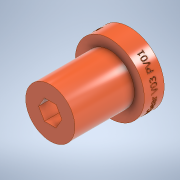
# Autodesk Inventor part: hexBushingForSideOppositeWormGear
Saved by Autodesk Inventor 2022.2 (Build 262287010, 287A)
## iProperties
Created: 2020-11-16
Part Number: hexBushingForSideOppositeWormGear
Material: PC/ABS Plastic
Document SubType Name: Modeling
Designer: robst
Density: 0.357273 g/cm^3
Appearance: Smooth - Light Orange
Author: robst
Autodesk Inventor part; units mm, degrees
(part 1 of 2)
ref_plane "YZ Plane" through (0, 0, 0) normal (1, 0, 0) x (0, 1, 0)
ref_plane "XY Plane" through (0, 0, 0) normal (0, 0, 1) x (1, 0, 0)
sketch "Sketch1" plane through (0, 0, 0) normal (0, 0, 1) x (1, 0, 0)
  line L0 (7.3323, 0) -> (3.6662, -6.35)
  line L1 (3.6662, -6.35) -> (-3.6662, -6.35)
  line L2 (-3.6662, -6.35) -> (-7.3323, 0)
  line L3 (-7.3323, 0) -> (-3.6662, 6.35)
  line L4 (-3.6662, 6.35) -> (3.6662, 6.35)
  line L5 (3.6662, 6.35) -> (7.3323, 0)
  point P0 (0, 0)
  point P1 (0, 0)
  dimension "d0" = 12.7
  constraints: 12 end point, 1 coincident, 1 horizontal, 13 other
  measures "d0" distance between parallel lines of L1 L4
extrude "Extrusion1" add sketch "Sketch1" along normal mid plane 25.4
sketch "Sketch2" plane through (0, 0, -12.7) normal (0, 0, -1) x (-1, 0, 0)
  circle A0 centre (0, 0) radius 15.748
  dimension "d3" = 31.496
  constraints: 1 centre point, 1 coincident
  measures "d3" diameter of A0
extrude "Extrusion2" add sketch "Sketch2" along normal blind 19.05
sketch "Sketch3" plane through (0, 0, -31.75) normal (0, 0, -1) x (-1, 0, 0)
  circle A0 centre (0, 0) radius 22.098
  dimension "d6" = 44.196
  constraints: 1 centre point, 1 coincident
  measures "d6" diameter of A0
extrude "Base" add sketch "Sketch3" along normal blind 12.7
sketch "Sketch6" plane through (-3.6662, 6.35, 12.7) normal (0, 1, 0) x (1, 0, 0)
  line L0 (7.3323, 0) -> (0, 0) construction
  line L1 (3.6662, 0) -> (3.6662, 34.6111) construction
  line L2 (19.4142, 25.4) -> (-12.0818, 25.4) projected
  point P0 (3.6662, 12.7)
  point P1 (3.6662, 19.2024)
  dimension "d13" = 6.1976
  constraints: 2 end point, 1 midpoint, 1 point on line, 1 vertical
  measures "d13" distance from line of point (3.666, 19.202) L2
hole "Hole1" at (0, 6.35, -6.5024) direction (0, -1, 0) diameter 4.318 end through all clearance for "Hex Machine Screw" size "#6" standard "Ansi Unified Screw Threads"
sketch "Sketch7" plane through (0, 0, 12.7) normal (0, 0, 1) x (1, 0, 0)
  point P0 (0, 0)
  point P1 (0, 0)
  constraints: 1 coincident
hole "Hole2" at (0, 0, 12.7) direction (0, 0, -1) diameter 6.3246 depth 7.874 counterbore diameter 6.604 counterbore depth 6.1239
ref_plane "Work Plane1" through (0, -22.098, -31.75) normal (0, 1, 0) x (-1, 0, 0)
sketch "Sketch8" plane through (0, -22.098, -31.75) normal (0, 1, 0) x (-1, 0, 0)
  line L0 (-22.098, -12.7) -> (22.098, -12.7) projected
  line L1 (-22.098, 0) -> (22.098, 0) projected
  line L2 (22.098, 0) -> (22.098, -12.7) construction
  line L3 (22.098, -6.35) -> (-22.098, -6.35) construction
  line L4 (-22.098, 0) -> (-22.098, -12.7) construction
  line L5 (53.7985, -8.255) -> (54.2802, -8.255)
  line L6 (54.2802, -8.255) -> (54.2802, -6.6248)
  spline S0 degree 2 poles (54.2802, -6.6248) (54.2802, -6.4272) (54.3172, -6.0876) (54.3728, -5.9857) knots 0 0 0 1 2 2 2
  spline S1 degree 2 poles (54.3728, -5.9857) (54.4314, -5.8776) (54.6414, -5.7726) (54.8205, -5.7726) knots 0 0 0 1 2 2 2
  spline S2 degree 2 poles (54.8205, -5.7726) (54.9995, -5.7726) (55.3793, -5.9641) (55.5615, -6.1184) knots 0 0 0 1 2 2 2
  line L7 (55.5615, -6.1184) -> (55.5615, -8.255)
  line L8 (55.5615, -8.255) -> (56.0431, -8.255)
  line L9 (56.0431, -8.255) -> (56.0431, -4.2752)
  line L10 (56.0431, -4.2752) -> (55.5615, -4.2752)
  line L11 (55.5615, -4.2752) -> (55.5615, -5.714)
  spline S3 degree 2 poles (55.5615, -5.714) (55.3453, -5.5195) (54.9285, -5.3157) (54.6939, -5.3157) knots 0 0 0 1 2 2 2
  spline S4 degree 2 poles (54.6939, -5.3157) (54.274, -5.3157) (53.7985, -5.8714) (53.7985, -6.3994) knots 0 0 0 1 2 2 2
  line L12 (53.7985, -6.3994) -> (53.7985, -8.255)
  spline S5 degree 2 poles (51.8811, -8.3198) (52.5666, -8.3198) (53.3199, -7.551) (53.3199, -6.8409) knots 0 0 0 1 2 2 2
  spline S6 degree 2 poles (53.3199, -6.8409) (53.3199, -6.1431) (52.5882, -5.3157) (51.9985, -5.3157) knots 0 0 0 1 2 2 2
  spline S7 degree 2 poles (51.9985, -5.3157) (51.7329, -5.3157) (51.3223, -5.4701) (51.171, -5.6337) knots 0 0 0 1 2 2 2
  spline S8 degree 2 poles (51.171, -5.6337) (51.0166, -5.7973) (50.853, -6.2697) (50.853, -6.6124) knots 0 0 0 1 2 2 2
  line L13 (50.853, -6.6124) -> (50.853, -6.8749)
  line L14 (50.853, -6.8749) -> (52.8321, -6.8749)
  spline S9 degree 2 poles (52.8321, -6.8749) (52.8321, -7.372) (52.3319, -7.8999) (51.8873, -7.8999) knots 0 0 0 1 2 2 2
  spline S10 degree 2 poles (51.8873, -7.8999) (51.7299, -7.8999) (51.4242, -7.8289) (51.3007, -7.7733) knots 0 0 0 1 2 2 2
  spline S11 degree 2 poles (51.3007, -7.7733) (51.171, -7.7116) (50.9919, -7.6035) (50.9333, -7.5541) knots 0 0 0 1 2 2 2
  line L15 (50.9333, -7.5541) -> (50.9055, -7.5541)
  line L16 (50.9055, -7.5541) -> (50.9055, -8.079)
  spline S12 degree 2 poles (50.9055, -8.079) (50.9889, -8.113) (51.242, -8.2118) (51.3408, -8.2396) knots 0 0 0 1 2 2 2
  spline S13 degree 2 poles (51.3408, -8.2396) (51.4798, -8.2797) (51.7082, -8.3198) (51.8811, -8.3198) knots 0 0 0 1 2 2 2
  spline S14 degree 2 poles (51.3223, -6.5075) (51.3285, -6.3129) (51.4088, -6.0289) (51.4859, -5.9332) knots 0 0 0 1 2 2 2
  spline S15 degree 2 poles (51.4859, -5.9332) (51.5693, -5.8251) (51.8317, -5.7109) (52.0263, -5.7109) knots 0 0 0 1 2 2 2
  spline S16 degree 2 poles (52.0263, -5.7109) (52.2177, -5.7109) (52.4863, -5.8251) (52.5975, -5.9363) knots 0 0 0 1 2 2 2
  spline S17 degree 2 poles (52.5975, -5.9363) (52.7055, -6.0505) (52.8167, -6.3253) (52.8321, -6.5075) knots 0 0 0 1 2 2 2
  line L17 (52.8321, -6.5075) -> (51.3223, -6.5075)
  line L18 (48.1452, -8.255) -> (48.735, -8.255)
  line L19 (48.735, -8.255) -> (49.4297, -7.1805)
  line L20 (49.4297, -7.1805) -> (50.1429, -8.255)
  line L21 (50.1429, -8.255) -> (50.6894, -8.255)
  line L22 (50.6894, -8.255) -> (49.6983, -6.8378)
  line L23 (49.6983, -6.8378) -> (50.6801, -5.396)
  line L24 (50.6801, -5.396) -> (50.0904, -5.396)
  line L25 (50.0904, -5.396) -> (49.3988, -6.4612)
  line L26 (49.3988, -6.4612) -> (48.6917, -5.396)
  line L27 (48.6917, -5.396) -> (48.1452, -5.396)
  line L28 (48.1452, -5.396) -> (49.1302, -6.807)
  line L29 (49.1302, -6.807) -> (48.1452, -8.255)
  spline S18 degree 2 poles (45.1504, -7.0848) (45.1504, -7.3689) (45.3665, -7.8042) (45.5456, -7.9462) knots 0 0 0 1 2 2 2
  spline S19 degree 2 poles (45.5456, -7.9462) (45.7617, -8.113) (46.2526, -8.255) (46.6416, -8.255) knots 0 0 0 1 2 2 2
  line L30 (46.6416, -8.255) -> (47.7346, -8.255)
  line L31 (47.7346, -8.255) -> (47.7346, -4.445)
  line L32 (47.7346, -4.445) -> (46.725, -4.445)
  spline S20 degree 2 poles (46.725, -4.445) (46.3174, -4.445) (45.9099, -4.4975) (45.7246, -4.5994) knots 0 0 0 1 2 2 2
  spline S21 degree 2 poles (45.7246, -4.5994) (45.5178, -4.7074) (45.3294, -5.0625) (45.3294, -5.3033) knots 0 0 0 1 2 2 2
  spline S22 degree 2 poles (45.3294, -5.3033) (45.3294, -5.5719) (45.6135, -5.998) (45.8636, -6.1184) knots 0 0 0 1 2 2 2
  line L33 (45.8636, -6.1184) -> (45.8636, -6.137)
  spline S23 degree 2 poles (45.8636, -6.137) (45.5239, -6.2296) (45.1504, -6.7205) (45.1504, -7.0848) knots 0 0 0 1 2 2 2
  spline S24 degree 2 poles (45.6783, -7.1064) (45.6783, -6.8903) (45.8018, -6.6124) (45.9871, -6.5136) knots 0 0 0 1 2 2 2
  spline S25 degree 2 poles (45.9871, -6.5136) (46.1075, -6.4519) (46.3915, -6.4148) (46.654, -6.4148) knots 0 0 0 1 2 2 2
  line L34 (46.654, -6.4148) -> (47.2283, -6.4148)
  line L35 (47.2283, -6.4148) -> (47.2283, -7.8227)
  line L36 (47.2283, -7.8227) -> (46.8176, -7.8227)
  spline S26 degree 2 poles (46.8176, -7.8227) (46.4842, -7.8227) (46.1013, -7.761) (45.9531, -7.6622) knots 0 0 0 1 2 2 2
  spline S27 degree 2 poles (45.9531, -7.6622) (45.8111, -7.5603) (45.6783, -7.3071) (45.6783, -7.1064) knots 0 0 0 1 2 2 2
  spline S28 degree 2 poles (45.8574, -5.3743) (45.8574, -5.2385) (45.95, -5.0347) (46.0519, -4.9761) knots 0 0 0 1 2 2 2
  spline S29 degree 2 poles (46.0519, -4.9761) (46.1754, -4.9081) (46.4749, -4.8773) (46.7435, -4.8773) knots 0 0 0 1 2 2 2
  line L37 (46.7435, -4.8773) -> (47.2283, -4.8773)
  line L38 (47.2283, -4.8773) -> (47.2283, -5.9918)
  line L39 (47.2283, -5.9918) -> (46.654, -5.9918)
  spline S30 degree 2 poles (46.654, -5.9918) (46.4162, -5.9918) (46.1908, -5.9424) (46.0704, -5.8653) knots 0 0 0 1 2 2 2
  spline S31 degree 2 poles (46.0704, -5.8653) (45.9531, -5.7912) (45.8574, -5.5534) (45.8574, -5.3743) knots 0 0 0 1 2 2 2
  line L40 (42.4611, -8.255) -> (42.9428, -8.255)
  line L41 (42.9428, -8.255) -> (42.9428, -7.9401)
  spline S32 degree 2 poles (42.9428, -7.9401) (43.1651, -8.1346) (43.5634, -8.3353) (43.8104, -8.3353) knots 0 0 0 1 2 2 2
  spline S33 degree 2 poles (43.8104, -8.3353) (43.9956, -8.3353) (44.326, -8.2118) (44.4464, -8.079) knots 0 0 0 1 2 2 2
  spline S34 degree 2 poles (44.4464, -8.079) (44.5699, -7.9462) (44.7058, -7.5418) (44.7058, -7.2516) knots 0 0 0 1 2 2 2
  line L42 (44.7058, -7.2516) -> (44.7058, -5.396)
  line L43 (44.7058, -5.396) -> (44.2241, -5.396)
  line L44 (44.2241, -5.396) -> (44.2241, -7.0262)
  spline S35 degree 2 poles (44.2241, -7.0262) (44.2241, -7.2546) (44.1901, -7.5541) (44.1315, -7.6653) knots 0 0 0 1 2 2 2
  spline S36 degree 2 poles (44.1315, -7.6653) (44.0728, -7.7764) (43.8721, -7.8783) (43.6838, -7.8783) knots 0 0 0 1 2 2 2
  spline S37 degree 2 poles (43.6838, -7.8783) (43.5078, -7.8783) (43.1095, -7.6776) (42.9428, -7.5325) knots 0 0 0 1 2 2 2
  line L45 (42.9428, -7.5325) -> (42.9428, -5.396)
  line L46 (42.9428, -5.396) -> (42.4611, -5.396)
  line L47 (42.4611, -5.396) -> (42.4611, -8.255)
  spline S38 degree 2 poles (40.9915, -8.3229) (41.2786, -8.3229) (41.7757, -8.1685) (41.9393, -8.0821) knots 0 0 0 1 2 2 2
  line L48 (41.9393, -8.0821) -> (41.9393, -7.5418)
  line L49 (41.9393, -7.5418) -> (41.9146, -7.5418)
  spline S39 degree 2 poles (41.9146, -7.5418) (41.8529, -7.5912) (41.6862, -7.7085) (41.5472, -7.7733) knots 0 0 0 1 2 2 2
  spline S40 degree 2 poles (41.5472, -7.7733) (41.4268, -7.832) (41.1304, -7.9185) (40.9729, -7.9185) knots 0 0 0 1 2 2 2
  spline S41 degree 2 poles (40.9729, -7.9185) (40.8587, -7.9185) (40.5963, -7.866) (40.5345, -7.8227) knots 0 0 0 1 2 2 2
  spline S42 degree 2 poles (40.5345, -7.8227) (40.445, -7.7641) (40.3647, -7.6313) (40.3647, -7.4955) knots 0 0 0 1 2 2 2
  spline S43 degree 2 poles (40.3647, -7.4955) (40.3647, -7.3257) (40.5499, -7.1497) (40.7877, -7.091) knots 0 0 0 1 2 2 2
  spline S44 degree 2 poles (40.7877, -7.091) (40.8803, -7.0694) (41.1767, -7.0076) (41.3033, -6.9737) knots 0 0 0 1 2 2 2
  spline S45 degree 2 poles (41.3033, -6.9737) (41.6306, -6.878) (41.927, -6.4828) (41.927, -6.2018) knots 0 0 0 1 2 2 2
  spline S46 degree 2 poles (41.927, -6.2018) (41.927, -5.8128) (41.3434, -5.328) (40.8618, -5.328) knots 0 0 0 1 2 2 2
  spline S47 degree 2 poles (40.8618, -5.328) (40.6241, -5.328) (40.1424, -5.4454) (39.9788, -5.5349) knots 0 0 0 1 2 2 2
  line L50 (39.9788, -5.5349) -> (39.9788, -6.0505)
  line L51 (39.9788, -6.0505) -> (40.0035, -6.0505)
  spline S48 degree 2 poles (40.0035, -6.0505) (40.1887, -5.9023) (40.6395, -5.7325) (40.8711, -5.7325) knots 0 0 0 1 2 2 2
  spline S49 degree 2 poles (40.8711, -5.7325) (41.1088, -5.7325) (41.4361, -5.9332) (41.4361, -6.1339) knots 0 0 0 1 2 2 2
  spline S50 degree 2 poles (41.4361, -6.1339) (41.4361, -6.316) (41.2416, -6.492) (41.0254, -6.5476) knots 0 0 0 1 2 2 2
  spline S51 degree 2 poles (41.0254, -6.5476) (40.9205, -6.5754) (40.6549, -6.631) (40.5098, -6.6649) knots 0 0 0 1 2 2 2
  spline S52 degree 2 poles (40.5098, -6.6649) (40.1949, -6.7452) (39.8738, -7.1126) (39.8738, -7.4306) knots 0 0 0 1 2 2 2
  spline S53 degree 2 poles (39.8738, -7.4306) (39.8738, -7.6159) (40.0189, -7.9432) (40.1609, -8.0636) knots 0 0 0 1 2 2 2
  spline S54 degree 2 poles (40.1609, -8.0636) (40.3122, -8.1902) (40.6982, -8.3229) (40.9915, -8.3229) knots 0 0 0 1 2 2 2
  line L52 (37.1815, -8.255) -> (37.6631, -8.255)
  line L53 (37.6631, -8.255) -> (37.6631, -6.6248)
  spline S55 degree 2 poles (37.6631, -6.6248) (37.6631, -6.4272) (37.7002, -6.0876) (37.7557, -5.9857) knots 0 0 0 1 2 2 2
  spline S56 degree 2 poles (37.7557, -5.9857) (37.8144, -5.8776) (38.0244, -5.7726) (38.2034, -5.7726) knots 0 0 0 1 2 2 2
  spline S57 degree 2 poles (38.2034, -5.7726) (38.3825, -5.7726) (38.7623, -5.9641) (38.9444, -6.1184) knots 0 0 0 1 2 2 2
  line L54 (38.9444, -6.1184) -> (38.9444, -8.255)
  line L55 (38.9444, -8.255) -> (39.4261, -8.255)
  line L56 (39.4261, -8.255) -> (39.4261, -4.2752)
  line L57 (39.4261, -4.2752) -> (38.9444, -4.2752)
  line L58 (38.9444, -4.2752) -> (38.9444, -5.714)
  spline S58 degree 2 poles (38.9444, -5.714) (38.7283, -5.5195) (38.3115, -5.3157) (38.0768, -5.3157) knots 0 0 0 1 2 2 2
  spline S59 degree 2 poles (38.0768, -5.3157) (37.6569, -5.3157) (37.1815, -5.8714) (37.1815, -6.3994) knots 0 0 0 1 2 2 2
  line L59 (37.1815, -6.3994) -> (37.1815, -8.255)
  line L60 (36.0144, -8.255) -> (36.496, -8.255)
  line L61 (36.496, -8.255) -> (36.496, -5.396)
  line L62 (36.496, -5.396) -> (36.0144, -5.396)
  line L63 (36.0144, -5.396) -> (36.0144, -8.255)
  line L64 (35.9804, -4.9205) -> (36.5269, -4.9205)
  line L65 (36.5269, -4.9205) -> (36.5269, -4.4203)
  line L66 (36.5269, -4.4203) -> (35.9804, -4.4203)
  line L67 (35.9804, -4.4203) -> (35.9804, -4.9205)
  line L68 (33.0627, -8.255) -> (33.5444, -8.255)
  line L69 (33.5444, -8.255) -> (33.5444, -6.6248)
  spline S60 degree 2 poles (33.5444, -6.6248) (33.5444, -6.4272) (33.5814, -6.0876) (33.637, -5.9857) knots 0 0 0 1 2 2 2
  spline S61 degree 2 poles (33.637, -5.9857) (33.6957, -5.8776) (33.9056, -5.7726) (34.0847, -5.7726) knots 0 0 0 1 2 2 2
  spline S62 degree 2 poles (34.0847, -5.7726) (34.2638, -5.7726) (34.6435, -5.9641) (34.8257, -6.1184) knots 0 0 0 1 2 2 2
  line L70 (34.8257, -6.1184) -> (34.8257, -8.255)
  line L71 (34.8257, -8.255) -> (35.3073, -8.255)
  line L72 (35.3073, -8.255) -> (35.3073, -5.396)
  line L73 (35.3073, -5.396) -> (34.8257, -5.396)
  line L74 (34.8257, -5.396) -> (34.8257, -5.714)
  spline S63 degree 2 poles (34.8257, -5.714) (34.6096, -5.5195) (34.1927, -5.3157) (33.9581, -5.3157) knots 0 0 0 1 2 2 2
  spline S64 degree 2 poles (33.9581, -5.3157) (33.5382, -5.3157) (33.0627, -5.8714) (33.0627, -6.3994) knots 0 0 0 1 2 2 2
  line L75 (33.0627, -6.3994) -> (33.0627, -8.255)
  spline S65 degree 2 poles (32.2847, -8.712) (32.2353, -8.7336) (32.0469, -8.8015) (31.9265, -8.8293) knots 0 0 0 1 2 2 2
  spline S66 degree 2 poles (31.9265, -8.8293) (31.7937, -8.8632) (31.5684, -8.9034) (31.4356, -8.9034) knots 0 0 0 1 2 2 2
  spline S67 degree 2 poles (31.4356, -8.9034) (31.2133, -8.9034) (30.9045, -8.7861) (30.8181, -8.6811) knots 0 0 0 1 2 2 2
  spline S68 degree 2 poles (30.8181, -8.6811) (30.7347, -8.5761) (30.6699, -8.3013) (30.6699, -8.1253) knots 0 0 0 1 2 2 2
  line L76 (30.6699, -8.1253) -> (30.6699, -7.8752)
  spline S69 degree 2 poles (30.6699, -7.8752) (30.8644, -8.045) (31.238, -8.2056) (31.519, -8.2056) knots 0 0 0 1 2 2 2
  spline S70 degree 2 poles (31.519, -8.2056) (32.0068, -8.2056) (32.5841, -7.48) (32.5841, -6.7977) knots 0 0 0 1 2 2 2
  spline S71 degree 2 poles (32.5841, -6.7977) (32.5841, -6.4426) (32.3835, -5.893) (32.2167, -5.6985) knots 0 0 0 1 2 2 2
  spline S72 degree 2 poles (32.2167, -5.6985) (32.0562, -5.5164) (31.6147, -5.3157) (31.38, -5.3157) knots 0 0 0 1 2 2 2
  spline S73 degree 2 poles (31.38, -5.3157) (31.1577, -5.3157) (30.8335, -5.4207) (30.6699, -5.5164) knots 0 0 0 1 2 2 2
  line L77 (30.6699, -5.5164) -> (30.6421, -5.396)
  line L78 (30.6421, -5.396) -> (30.1882, -5.396)
  line L79 (30.1882, -5.396) -> (30.1882, -7.9277)
  spline S74 degree 2 poles (30.1882, -7.9277) (30.1882, -8.6564) (30.8212, -9.3356) (31.4726, -9.3356) knots 0 0 0 1 2 2 2
  spline S75 degree 2 poles (31.4726, -9.3356) (31.6826, -9.3356) (32.121, -9.2677) (32.3094, -9.2121) knots 0 0 0 1 2 2 2
  line L80 (32.3094, -9.2121) -> (32.3094, -8.712)
  line L81 (32.3094, -8.712) -> (32.2847, -8.712)
  line L82 (30.6699, -7.48) -> (30.6699, -5.9085)
  spline S76 degree 2 poles (30.6699, -5.9085) (30.849, -5.822) (31.1515, -5.7479) (31.3028, -5.7479) knots 0 0 0 1 2 2 2
  spline S77 degree 2 poles (31.3028, -5.7479) (31.6672, -5.7479) (32.0871, -6.2852) (32.0871, -6.7884) knots 0 0 0 1 2 2 2
  spline S78 degree 2 poles (32.0871, -6.7884) (32.0871, -7.2639) (31.769, -7.761) (31.4109, -7.761) knots 0 0 0 1 2 2 2
  spline S79 degree 2 poles (31.4109, -7.761) (31.2226, -7.761) (30.8273, -7.6128) (30.6699, -7.48) knots 0 0 0 1 2 2 2
  line L83 (27.1748, -4.8958) -> (28.947, -4.8958)
  line L84 (28.947, -4.8958) -> (28.947, -5.9702)
  line L85 (28.947, -5.9702) -> (27.2489, -5.9702)
  line L86 (27.2489, -5.9702) -> (27.2489, -6.421)
  line L87 (27.2489, -6.421) -> (28.947, -6.421)
  line L88 (28.947, -6.421) -> (28.947, -8.255)
  line L89 (28.947, -8.255) -> (29.4534, -8.255)
  line L90 (29.4534, -8.255) -> (29.4534, -4.445)
  line L91 (29.4534, -4.445) -> (27.1748, -4.445)
  line L92 (27.1748, -4.445) -> (27.1748, -4.8958)
  spline S80 degree 2 poles (24.4084, -6.8255) (24.4084, -7.548) (25.1031, -8.3353) (25.6835, -8.3353) knots 0 0 0 1 2 2 2
  spline S81 degree 2 poles (25.6835, -8.3353) (26.2794, -8.3353) (26.9618, -7.5233) (26.9618, -6.8255) knots 0 0 0 1 2 2 2
  spline S82 degree 2 poles (26.9618, -6.8255) (26.9618, -6.1092) (26.2578, -5.3157) (25.6835, -5.3157) knots 0 0 0 1 2 2 2
  spline S83 degree 2 poles (25.6835, -5.3157) (25.1031, -5.3157) (24.4084, -6.1061) (24.4084, -6.8255) knots 0 0 0 1 2 2 2
  spline S84 degree 2 poles (24.9055, -6.8255) (24.9055, -6.2697) (25.3099, -5.7294) (25.6835, -5.7294) knots 0 0 0 1 2 2 2
  spline S85 degree 2 poles (25.6835, -5.7294) (26.0571, -5.7294) (26.4647, -6.2697) (26.4647, -6.8255) knots 0 0 0 1 2 2 2
  spline S86 degree 2 poles (26.4647, -6.8255) (26.4647, -7.3658) (26.0571, -7.9215) (25.6835, -7.9215) knots 0 0 0 1 2 2 2
  spline S87 degree 2 poles (25.6835, -7.9215) (25.313, -7.9215) (24.9055, -7.3751) (24.9055, -6.8255) knots 0 0 0 1 2 2 2
  line L93 (22.3984, -5.9116) -> (22.4231, -5.9116)
  spline S88 degree 2 poles (22.4231, -5.9116) (22.4787, -5.8961) (22.5991, -5.89) (22.6825, -5.89) knots 0 0 0 1 2 2 2
  spline S89 degree 2 poles (22.6825, -5.89) (22.877, -5.89) (23.2598, -6.0598) (23.4327, -6.2265) knots 0 0 0 1 2 2 2
  line L94 (23.4327, -6.2265) -> (23.4327, -8.255)
  line L95 (23.4327, -8.255) -> (23.9144, -8.255)
  line L96 (23.9144, -8.255) -> (23.9144, -5.396)
  line L97 (23.9144, -5.396) -> (23.4327, -5.396)
  line L98 (23.4327, -5.396) -> (23.4327, -5.822)
  spline S90 degree 2 poles (23.4327, -5.822) (23.1703, -5.5874) (22.7782, -5.396) (22.5929, -5.396) knots 0 0 0 1 2 2 2
  spline S91 degree 2 poles (22.5929, -5.396) (22.5188, -5.396) (22.4447, -5.4021) (22.3984, -5.4114) knots 0 0 0 1 2 2 2
  line L99 (22.3984, -5.4114) -> (22.3984, -5.9116)
  spline S92 degree 2 poles (19.2924, -4.8803) (19.0762, -5.1335) (18.8354, -5.8745) (18.8354, -6.35) knots 0 0 0 1 2 2 2
  spline S93 degree 2 poles (18.8354, -6.35) (18.8354, -6.8131) (19.0701, -7.5634) (19.2924, -7.8166) knots 0 0 0 1 2 2 2
  spline S94 degree 2 poles (19.2924, -7.8166) (19.527, -8.0821) (20.1476, -8.3353) (20.5212, -8.3353) knots 0 0 0 1 2 2 2
  spline S95 degree 2 poles (20.5212, -8.3353) (20.9071, -8.3353) (21.5246, -8.0728) (21.75, -7.8166) knots 0 0 0 1 2 2 2
  spline S96 degree 2 poles (21.75, -7.8166) (21.9693, -7.5634) (22.2039, -6.8193) (22.2039, -6.35) knots 0 0 0 1 2 2 2
  spline S97 degree 2 poles (22.2039, -6.35) (22.2039, -5.8714) (21.9662, -5.1428) (21.747, -4.8803) knots 0 0 0 1 2 2 2
  spline S98 degree 2 poles (21.747, -4.8803) (21.5246, -4.6272) (20.9041, -4.3647) (20.5212, -4.3647) knots 0 0 0 1 2 2 2
  spline S99 degree 2 poles (20.5212, -4.3647) (20.1322, -4.3647) (19.5085, -4.6364) (19.2924, -4.8803) knots 0 0 0 1 2 2 2
  spline S100 degree 2 poles (19.3634, -6.35) (19.3634, -5.9733) (19.527, -5.3898) (19.6752, -5.1984) knots 0 0 0 1 2 2 2
  spline S101 degree 2 poles (19.6752, -5.1984) (19.8265, -5.0008) (20.2526, -4.8032) (20.5181, -4.8032) knots 0 0 0 1 2 2 2
  spline S102 degree 2 poles (20.5181, -4.8032) (20.7929, -4.8032) (21.2066, -4.9946) (21.3641, -5.1984) knots 0 0 0 1 2 2 2
  spline S103 degree 2 poles (21.3641, -5.1984) (21.5154, -5.3929) (21.6759, -5.9795) (21.6759, -6.35) knots 0 0 0 1 2 2 2
  spline S104 degree 2 poles (21.6759, -6.35) (21.6759, -7.1003) (21.0461, -7.8968) (20.5181, -7.8968) knots 0 0 0 1 2 2 2
  spline S105 degree 2 poles (20.5181, -7.8968) (19.9902, -7.8968) (19.3634, -7.1003) (19.3634, -6.35) knots 0 0 0 1 2 2 2
  spline S106 degree 2 poles (15.9208, -6.7483) (15.9208, -7.4646) (16.6031, -8.3106) (17.1249, -8.3106) knots 0 0 0 1 2 2 2
  spline S107 degree 2 poles (17.1249, -8.3106) (17.338, -8.3106) (17.6652, -8.2118) (17.8351, -8.1099) knots 0 0 0 1 2 2 2
  line L100 (17.8351, -8.1099) -> (17.8351, -9.3078)
  line L101 (17.8351, -9.3078) -> (18.3167, -9.3078)
  line L102 (18.3167, -9.3078) -> (18.3167, -5.396)
  line L103 (18.3167, -5.396) -> (17.8351, -5.396)
  line L104 (17.8351, -5.396) -> (17.8351, -5.6954)
  spline S108 degree 2 poles (17.8351, -5.6954) (17.656, -5.5318) (17.2176, -5.3157) (16.9613, -5.3157) knots 0 0 0 1 2 2 2
  spline S109 degree 2 poles (16.9613, -5.3157) (16.4704, -5.3157) (15.9208, -6.0937) (15.9208, -6.7483) knots 0 0 0 1 2 2 2
  spline S110 degree 2 poles (16.4179, -6.8039) (16.4179, -6.3129) (16.7297, -5.7726) (17.0786, -5.7726) knots 0 0 0 1 2 2 2
  spline S111 degree 2 poles (17.0786, -5.7726) (17.2824, -5.7726) (17.6652, -5.9548) (17.8351, -6.0968) knots 0 0 0 1 2 2 2
  line L105 (17.8351, -6.0968) -> (17.8351, -7.7209)
  spline S112 degree 2 poles (17.8351, -7.7209) (17.6467, -7.8104) (17.3781, -7.8783) (17.2052, -7.8783) knots 0 0 0 1 2 2 2
  spline S113 degree 2 poles (17.2052, -7.8783) (16.8316, -7.8783) (16.4179, -7.3287) (16.4179, -6.8039) knots 0 0 0 1 2 2 2
  spline S114 degree 2 poles (13.0247, -6.7483) (13.0247, -7.4646) (13.707, -8.3106) (14.2288, -8.3106) knots 0 0 0 1 2 2 2
  spline S115 degree 2 poles (14.2288, -8.3106) (14.4419, -8.3106) (14.7692, -8.2118) (14.939, -8.1099) knots 0 0 0 1 2 2 2
  line L106 (14.939, -8.1099) -> (14.939, -9.3078)
  line L107 (14.939, -9.3078) -> (15.4206, -9.3078)
  line L108 (15.4206, -9.3078) -> (15.4206, -5.396)
  line L109 (15.4206, -5.396) -> (14.939, -5.396)
  line L110 (14.939, -5.396) -> (14.939, -5.6954)
  spline S116 degree 2 poles (14.939, -5.6954) (14.7599, -5.5318) (14.3215, -5.3157) (14.0652, -5.3157) knots 0 0 0 1 2 2 2
  spline S117 degree 2 poles (14.0652, -5.3157) (13.5743, -5.3157) (13.0247, -6.0937) (13.0247, -6.7483) knots 0 0 0 1 2 2 2
  spline S118 degree 2 poles (13.5218, -6.8039) (13.5218, -6.3129) (13.8336, -5.7726) (14.1825, -5.7726) knots 0 0 0 1 2 2 2
  spline S119 degree 2 poles (14.1825, -5.7726) (14.3863, -5.7726) (14.7692, -5.9548) (14.939, -6.0968) knots 0 0 0 1 2 2 2
  line L111 (14.939, -6.0968) -> (14.939, -7.7209)
  spline S120 degree 2 poles (14.939, -7.7209) (14.7506, -7.8104) (14.482, -7.8783) (14.3091, -7.8783) knots 0 0 0 1 2 2 2
  spline S121 degree 2 poles (14.3091, -7.8783) (13.9355, -7.8783) (13.5218, -7.3287) (13.5218, -6.8039) knots 0 0 0 1 2 2 2
  spline S122 degree 2 poles (10.1749, -6.8255) (10.1749, -7.548) (10.8696, -8.3353) (11.4501, -8.3353) knots 0 0 0 1 2 2 2
  spline S123 degree 2 poles (11.4501, -8.3353) (12.046, -8.3353) (12.7283, -7.5233) (12.7283, -6.8255) knots 0 0 0 1 2 2 2
  spline S124 degree 2 poles (12.7283, -6.8255) (12.7283, -6.1092) (12.0243, -5.3157) (11.4501, -5.3157) knots 0 0 0 1 2 2 2
  spline S125 degree 2 poles (11.4501, -5.3157) (10.8696, -5.3157) (10.1749, -6.1061) (10.1749, -6.8255) knots 0 0 0 1 2 2 2
  spline S126 degree 2 poles (10.672, -6.8255) (10.672, -6.2697) (11.0765, -5.7294) (11.4501, -5.7294) knots 0 0 0 1 2 2 2
  spline S127 degree 2 poles (11.4501, -5.7294) (11.8237, -5.7294) (12.2312, -6.2697) (12.2312, -6.8255) knots 0 0 0 1 2 2 2
  spline S128 degree 2 poles (12.2312, -6.8255) (12.2312, -7.3658) (11.8237, -7.9215) (11.4501, -7.9215) knots 0 0 0 1 2 2 2
  spline S129 degree 2 poles (11.4501, -7.9215) (11.0796, -7.9215) (10.672, -7.3751) (10.672, -6.8255) knots 0 0 0 1 2 2 2
  spline S130 degree 2 poles (8.909, -8.3229) (9.1962, -8.3229) (9.6933, -8.1685) (9.8569, -8.0821) knots 0 0 0 1 2 2 2
  line L112 (9.8569, -8.0821) -> (9.8569, -7.5418)
  line L113 (9.8569, -7.5418) -> (9.8322, -7.5418)
  spline S131 degree 2 poles (9.8322, -7.5418) (9.7705, -7.5912) (9.6037, -7.7085) (9.4648, -7.7733) knots 0 0 0 1 2 2 2
  spline S132 degree 2 poles (9.4648, -7.7733) (9.3444, -7.832) (9.048, -7.9185) (8.8905, -7.9185) knots 0 0 0 1 2 2 2
  spline S133 degree 2 poles (8.8905, -7.9185) (8.7763, -7.9185) (8.5138, -7.866) (8.4521, -7.8227) knots 0 0 0 1 2 2 2
  spline S134 degree 2 poles (8.4521, -7.8227) (8.3626, -7.7641) (8.2823, -7.6313) (8.2823, -7.4955) knots 0 0 0 1 2 2 2
  spline S135 degree 2 poles (8.2823, -7.4955) (8.2823, -7.3257) (8.4675, -7.1497) (8.7053, -7.091) knots 0 0 0 1 2 2 2
  spline S136 degree 2 poles (8.7053, -7.091) (8.7979, -7.0694) (9.0943, -7.0076) (9.2209, -6.9737) knots 0 0 0 1 2 2 2
  spline S137 degree 2 poles (9.2209, -6.9737) (9.5482, -6.878) (9.8446, -6.4828) (9.8446, -6.2018) knots 0 0 0 1 2 2 2
  spline S138 degree 2 poles (9.8446, -6.2018) (9.8446, -5.8128) (9.261, -5.328) (8.7794, -5.328) knots 0 0 0 1 2 2 2
  spline S139 degree 2 poles (8.7794, -5.328) (8.5416, -5.328) (8.06, -5.4454) (7.8963, -5.5349) knots 0 0 0 1 2 2 2
  line L114 (7.8963, -5.5349) -> (7.8963, -6.0505)
  line L115 (7.8963, -6.0505) -> (7.921, -6.0505)
  spline S140 degree 2 poles (7.921, -6.0505) (8.1063, -5.9023) (8.5571, -5.7325) (8.7886, -5.7325) knots 0 0 0 1 2 2 2
  spline S141 degree 2 poles (8.7886, -5.7325) (9.0264, -5.7325) (9.3536, -5.9332) (9.3536, -6.1339) knots 0 0 0 1 2 2 2
  spline S142 degree 2 poles (9.3536, -6.1339) (9.3536, -6.316) (9.1591, -6.492) (8.943, -6.5476) knots 0 0 0 1 2 2 2
  spline S143 degree 2 poles (8.943, -6.5476) (8.838, -6.5754) (8.5725, -6.631) (8.4274, -6.6649) knots 0 0 0 1 2 2 2
  spline S144 degree 2 poles (8.4274, -6.6649) (8.1125, -6.7452) (7.7914, -7.1126) (7.7914, -7.4306) knots 0 0 0 1 2 2 2
  spline S145 degree 2 poles (7.7914, -7.4306) (7.7914, -7.6159) (7.9365, -7.9432) (8.0785, -8.0636) knots 0 0 0 1 2 2 2
  spline S146 degree 2 poles (8.0785, -8.0636) (8.2298, -8.1902) (8.6157, -8.3229) (8.909, -8.3229) knots 0 0 0 1 2 2 2
  line L116 (6.8528, -8.255) -> (7.3344, -8.255)
  line L117 (7.3344, -8.255) -> (7.3344, -5.396)
  line L118 (7.3344, -5.396) -> (6.8528, -5.396)
  line L119 (6.8528, -5.396) -> (6.8528, -8.255)
  line L120 (6.8188, -4.9205) -> (7.3653, -4.9205)
  line L121 (7.3653, -4.9205) -> (7.3653, -4.4203)
  line L122 (7.3653, -4.4203) -> (6.8188, -4.4203)
  line L123 (6.8188, -4.4203) -> (6.8188, -4.9205)
  spline S147 degree 2 poles (5.2812, -8.3106) (5.6733, -8.3106) (6.1148, -7.8629) (6.1148, -7.3781) knots 0 0 0 1 2 2 2
  line L124 (6.1148, -7.3781) -> (6.1148, -5.7942)
  line L125 (6.1148, -5.7942) -> (6.439, -5.7942)
  line L126 (6.439, -5.7942) -> (6.439, -5.396)
  line L127 (6.439, -5.396) -> (6.1148, -5.396)
  line L128 (6.1148, -5.396) -> (6.1148, -4.5747)
  line L129 (6.1148, -4.5747) -> (5.6332, -4.5747)
  line L130 (5.6332, -4.5747) -> (5.6332, -5.396)
  line L131 (5.6332, -5.396) -> (4.7471, -5.396)
  line L132 (4.7471, -5.396) -> (4.7471, -5.7942)
  line L133 (4.7471, -5.7942) -> (5.6332, -5.7942)
  line L134 (5.6332, -5.7942) -> (5.6332, -7.1558)
  spline S148 degree 2 poles (5.6332, -7.1558) (5.6332, -7.372) (5.6177, -7.6097) (5.5653, -7.7116) knots 0 0 0 1 2 2 2
  spline S149 degree 2 poles (5.5653, -7.7116) (5.522, -7.8011) (5.3275, -7.8907) (5.1608, -7.8907) knots 0 0 0 1 2 2 2
  spline S150 degree 2 poles (5.1608, -7.8907) (5.0435, -7.8907) (4.8243, -7.8197) (4.7749, -7.798) knots 0 0 0 1 2 2 2
  line L135 (4.7749, -7.798) -> (4.7471, -7.798)
  line L136 (4.7471, -7.798) -> (4.7471, -8.2303)
  spline S151 degree 2 poles (4.7471, -8.2303) (4.8829, -8.2674) (5.1608, -8.3106) (5.2812, -8.3106) knots 0 0 0 1 2 2 2
  spline S152 degree 2 poles (3.1508, -8.3198) (3.8362, -8.3198) (4.5896, -7.551) (4.5896, -6.8409) knots 0 0 0 1 2 2 2
  spline S153 degree 2 poles (4.5896, -6.8409) (4.5896, -6.1431) (3.8579, -5.3157) (3.2681, -5.3157) knots 0 0 0 1 2 2 2
  spline S154 degree 2 poles (3.2681, -5.3157) (3.0026, -5.3157) (2.592, -5.4701) (2.4407, -5.6337) knots 0 0 0 1 2 2 2
  spline S155 degree 2 poles (2.4407, -5.6337) (2.2863, -5.7973) (2.1227, -6.2697) (2.1227, -6.6124) knots 0 0 0 1 2 2 2
  line L137 (2.1227, -6.6124) -> (2.1227, -6.8749)
  line L138 (2.1227, -6.8749) -> (4.1018, -6.8749)
  spline S156 degree 2 poles (4.1018, -6.8749) (4.1018, -7.372) (3.6016, -7.8999) (3.157, -7.8999) knots 0 0 0 1 2 2 2
  spline S157 degree 2 poles (3.157, -7.8999) (2.9995, -7.8999) (2.6939, -7.8289) (2.5704, -7.7733) knots 0 0 0 1 2 2 2
  spline S158 degree 2 poles (2.5704, -7.7733) (2.4407, -7.7116) (2.2616, -7.6035) (2.2029, -7.5541) knots 0 0 0 1 2 2 2
  line L139 (2.2029, -7.5541) -> (2.1752, -7.5541)
  line L140 (2.1752, -7.5541) -> (2.1752, -8.079)
  spline S159 degree 2 poles (2.1752, -8.079) (2.2585, -8.113) (2.5117, -8.2118) (2.6105, -8.2396) knots 0 0 0 1 2 2 2
  spline S160 degree 2 poles (2.6105, -8.2396) (2.7494, -8.2797) (2.9779, -8.3198) (3.1508, -8.3198) knots 0 0 0 1 2 2 2
  spline S161 degree 2 poles (2.592, -6.5075) (2.5982, -6.3129) (2.6784, -6.0289) (2.7556, -5.9332) knots 0 0 0 1 2 2 2
  spline S162 degree 2 poles (2.7556, -5.9332) (2.839, -5.8251) (3.1014, -5.7109) (3.2959, -5.7109) knots 0 0 0 1 2 2 2
  spline S163 degree 2 poles (3.2959, -5.7109) (3.4874, -5.7109) (3.756, -5.8251) (3.8671, -5.9363) knots 0 0 0 1 2 2 2
  spline S164 degree 2 poles (3.8671, -5.9363) (3.9752, -6.0505) (4.0863, -6.3253) (4.1018, -6.5075) knots 0 0 0 1 2 2 2
  line L141 (4.1018, -6.5075) -> (2.592, -6.5075)
  spline S165 degree 2 poles (0.5357, -8.3229) (0.9494, -8.3229) (1.5299, -8.15) (1.7861, -8.0265) knots 0 0 0 1 2 2 2
  line L142 (1.7861, -8.0265) -> (1.7861, -7.3905)
  line L143 (1.7861, -7.3905) -> (1.7491, -7.3905)
  spline S166 degree 2 poles (1.7491, -7.3905) (1.499, -7.6251) (0.8661, -7.8845) (0.5727, -7.8845) knots 0 0 0 1 2 2 2
  spline S167 degree 2 poles (0.5727, -7.8845) (0.1528, -7.8845) (-0.2763, -7.5356) (-0.2763, -7.2485) knots 0 0 0 1 2 2 2
  spline S168 degree 2 poles (-0.2763, -7.2485) (-0.2763, -7.02) (-0.0509, -6.7359) (0.193, -6.6649) knots 0 0 0 1 2 2 2
  spline S169 degree 2 poles (0.193, -6.6649) (0.369, -6.6155) (0.6623, -6.5476) (0.8815, -6.492) knots 0 0 0 1 2 2 2
  spline S170 degree 2 poles (0.8815, -6.492) (1.0791, -6.4395) (1.3909, -6.2821) (1.5113, -6.1555) knots 0 0 0 1 2 2 2
  spline S171 degree 2 poles (1.5113, -6.1555) (1.6287, -6.0289) (1.7583, -5.6893) (1.7583, -5.467) knots 0 0 0 1 2 2 2
  spline S172 degree 2 poles (1.7583, -5.467) (1.7583, -5.0038) (1.0359, -4.3771) (0.477, -4.3771) knots 0 0 0 1 2 2 2
  spline S173 degree 2 poles (0.477, -4.3771) (0.1559, -4.3771) (-0.4122, -4.5037) (-0.6561, -4.6241) knots 0 0 0 1 2 2 2
  line L144 (-0.6561, -4.6241) -> (-0.6561, -5.2292)
  line L145 (-0.6561, -5.2292) -> (-0.619, -5.2292)
  spline S174 degree 2 poles (-0.619, -5.2292) (-0.4369, -5.0625) (0.1312, -4.8155) (0.4431, -4.8155) knots 0 0 0 1 2 2 2
  spline S175 degree 2 poles (0.4431, -4.8155) (0.795, -4.8155) (1.2304, -5.1459) (1.2304, -5.4145) knots 0 0 0 1 2 2 2
  spline S176 degree 2 poles (1.2304, -5.4145) (1.2304, -5.6553) (0.9741, -5.9424) (0.7333, -6.0073) knots 0 0 0 1 2 2 2
  spline S177 degree 2 poles (0.7333, -6.0073) (0.5727, -6.0505) (0.1065, -6.1617) (-0.0479, -6.208) knots 0 0 0 1 2 2 2
  spline S178 degree 2 poles (-0.0479, -6.208) (-0.44, -6.3284) (-0.8043, -6.8131) (-0.8043, -7.1682) knots 0 0 0 1 2 2 2
  spline S179 degree 2 poles (-0.8043, -7.1682) (-0.8043, -7.3936) (-0.6221, -7.8258) (-0.4585, -7.9771) knots 0 0 0 1 2 2 2
  spline S180 degree 2 poles (-0.4585, -7.9771) (-0.2763, -8.1438) (0.1868, -8.3229) (0.5357, -8.3229) knots 0 0 0 1 2 2 2
  line L146 (-1.7738, -8.255) -> (-1.2921, -8.255)
  line L147 (-1.2921, -8.255) -> (-1.2921, -5.396)
  line L148 (-1.2921, -5.396) -> (-1.7738, -5.396)
  line L149 (-1.7738, -5.396) -> (-1.7738, -8.255)
  line L150 (-1.8077, -4.9205) -> (-1.2613, -4.9205)
  line L151 (-1.2613, -4.9205) -> (-1.2613, -4.4203)
  line L152 (-1.2613, -4.4203) -> (-1.8077, -4.4203)
  line L153 (-1.8077, -4.4203) -> (-1.8077, -4.9205)
  line L154 (-4.6791, -8.255) -> (-4.1975, -8.255)
  line L155 (-4.1975, -8.255) -> (-4.1975, -7.9648)
  spline S181 degree 2 poles (-4.1975, -7.9648) (-4.0863, -8.0574) (-3.9227, -8.1809) (-3.8115, -8.2334) knots 0 0 0 1 2 2 2
  spline S182 degree 2 poles (-3.8115, -8.2334) (-3.7097, -8.2828) (-3.4904, -8.3353) (-3.3453, -8.3353) knots 0 0 0 1 2 2 2
  spline S183 degree 2 poles (-3.3453, -8.3353) (-3.1107, -8.3353) (-2.7155, -8.1408) (-2.5765, -7.9524) knots 0 0 0 1 2 2 2
  spline S184 degree 2 poles (-2.5765, -7.9524) (-2.4376, -7.7641) (-2.2832, -7.2083) (-2.2832, -6.8471) knots 0 0 0 1 2 2 2
  spline S185 degree 2 poles (-2.2832, -6.8471) (-2.2832, -6.4704) (-2.4777, -5.9208) (-2.6475, -5.714) knots 0 0 0 1 2 2 2
  spline S186 degree 2 poles (-2.6475, -5.714) (-2.805, -5.5287) (-3.2465, -5.3157) (-3.4904, -5.3157) knots 0 0 0 1 2 2 2
  spline S187 degree 2 poles (-3.4904, -5.3157) (-3.7035, -5.3157) (-4.0215, -5.4114) (-4.1975, -5.5102) knots 0 0 0 1 2 2 2
  line L156 (-4.1975, -5.5102) -> (-4.1975, -4.2752)
  line L157 (-4.1975, -4.2752) -> (-4.6791, -4.2752)
  line L158 (-4.6791, -4.2752) -> (-4.6791, -8.255)
  line L159 (-4.1975, -7.5603) -> (-4.1975, -5.9085)
  spline S188 degree 2 poles (-4.1975, -5.9085) (-4.0184, -5.822) (-3.7344, -5.7572) (-3.5707, -5.7572) knots 0 0 0 1 2 2 2
  spline S189 degree 2 poles (-3.5707, -5.7572) (-3.2002, -5.7572) (-2.7803, -6.3129) (-2.7803, -6.8378) knots 0 0 0 1 2 2 2
  spline S190 degree 2 poles (-2.7803, -6.8378) (-2.7803, -7.3442) (-3.1014, -7.8783) (-3.4565, -7.8783) knots 0 0 0 1 2 2 2
  spline S191 degree 2 poles (-3.4565, -7.8783) (-3.6448, -7.8783) (-4.0277, -7.7054) (-4.1975, -7.5603) knots 0 0 0 1 2 2 2
  spline S192 degree 2 poles (-6.6181, -8.3198) (-5.9327, -8.3198) (-5.1793, -7.551) (-5.1793, -6.8409) knots 0 0 0 1 2 2 2
  spline S193 degree 2 poles (-5.1793, -6.8409) (-5.1793, -6.1431) (-5.9111, -5.3157) (-6.5008, -5.3157) knots 0 0 0 1 2 2 2
  spline S194 degree 2 poles (-6.5008, -5.3157) (-6.7663, -5.3157) (-7.1769, -5.4701) (-7.3282, -5.6337) knots 0 0 0 1 2 2 2
  spline S195 degree 2 poles (-7.3282, -5.6337) (-7.4826, -5.7973) (-7.6462, -6.2697) (-7.6462, -6.6124) knots 0 0 0 1 2 2 2
  line L160 (-7.6462, -6.6124) -> (-7.6462, -6.8749)
  line L161 (-7.6462, -6.8749) -> (-5.6671, -6.8749)
  spline S196 degree 2 poles (-5.6671, -6.8749) (-5.6671, -7.372) (-6.1673, -7.8999) (-6.6119, -7.8999) knots 0 0 0 1 2 2 2
  spline S197 degree 2 poles (-6.6119, -7.8999) (-6.7694, -7.8999) (-7.0751, -7.8289) (-7.1986, -7.7733) knots 0 0 0 1 2 2 2
  spline S198 degree 2 poles (-7.1986, -7.7733) (-7.3282, -7.7116) (-7.5073, -7.6035) (-7.566, -7.5541) knots 0 0 0 1 2 2 2
  line L162 (-7.566, -7.5541) -> (-7.5938, -7.5541)
  line L163 (-7.5938, -7.5541) -> (-7.5938, -8.079)
  spline S199 degree 2 poles (-7.5938, -8.079) (-7.5104, -8.113) (-7.2572, -8.2118) (-7.1584, -8.2396) knots 0 0 0 1 2 2 2
  spline S200 degree 2 poles (-7.1584, -8.2396) (-7.0195, -8.2797) (-6.791, -8.3198) (-6.6181, -8.3198) knots 0 0 0 1 2 2 2
  spline S201 degree 2 poles (-7.1769, -6.5075) (-7.1708, -6.3129) (-7.0905, -6.0289) (-7.0133, -5.9332) knots 0 0 0 1 2 2 2
  spline S202 degree 2 poles (-7.0133, -5.9332) (-6.9299, -5.8251) (-6.6675, -5.7109) (-6.473, -5.7109) knots 0 0 0 1 2 2 2
  spline S203 degree 2 poles (-6.473, -5.7109) (-6.2816, -5.7109) (-6.0129, -5.8251) (-5.9018, -5.9363) knots 0 0 0 1 2 2 2
  spline S204 degree 2 poles (-5.9018, -5.9363) (-5.7937, -6.0505) (-5.6826, -6.3253) (-5.6671, -6.5075) knots 0 0 0 1 2 2 2
  line L164 (-5.6671, -6.5075) -> (-7.1769, -6.5075)
  line L165 (-12.4412, -4.445) -> (-11.484, -8.255)
  line L166 (-11.484, -8.255) -> (-10.9159, -8.255)
  line L167 (-10.9159, -8.255) -> (-10.141, -5.0934)
  line L168 (-10.141, -5.0934) -> (-9.3876, -8.255)
  line L169 (-9.3876, -8.255) -> (-8.8257, -8.255)
  line L170 (-8.8257, -8.255) -> (-7.8531, -4.445)
  line L171 (-7.8531, -4.445) -> (-8.3749, -4.445)
  line L172 (-8.3749, -4.445) -> (-9.1406, -7.6035)
  line L173 (-9.1406, -7.6035) -> (-9.9001, -4.445)
  line L174 (-9.9001, -4.445) -> (-10.4157, -4.445)
  line L175 (-10.4157, -4.445) -> (-11.1815, -7.6406)
  line L176 (-11.1815, -7.6406) -> (-11.9441, -4.445)
  line L177 (-11.9441, -4.445) -> (-12.4412, -4.445)
  spline S205 degree 2 poles (-15.2076, -6.8255) (-15.2076, -7.548) (-14.5129, -8.3353) (-13.9324, -8.3353) knots 0 0 0 1 2 2 2
  spline S206 degree 2 poles (-13.9324, -8.3353) (-13.3365, -8.3353) (-12.6542, -7.5233) (-12.6542, -6.8255) knots 0 0 0 1 2 2 2
  spline S207 degree 2 poles (-12.6542, -6.8255) (-12.6542, -6.1092) (-13.3582, -5.3157) (-13.9324, -5.3157) knots 0 0 0 1 2 2 2
  spline S208 degree 2 poles (-13.9324, -5.3157) (-14.5129, -5.3157) (-15.2076, -6.1061) (-15.2076, -6.8255) knots 0 0 0 1 2 2 2
  spline S209 degree 2 poles (-14.7105, -6.8255) (-14.7105, -6.2697) (-14.306, -5.7294) (-13.9324, -5.7294) knots 0 0 0 1 2 2 2
  spline S210 degree 2 poles (-13.9324, -5.7294) (-13.5588, -5.7294) (-13.1513, -6.2697) (-13.1513, -6.8255) knots 0 0 0 1 2 2 2
  spline S211 degree 2 poles (-13.1513, -6.8255) (-13.1513, -7.3658) (-13.5588, -7.9215) (-13.9324, -7.9215) knots 0 0 0 1 2 2 2
  spline S212 degree 2 poles (-13.9324, -7.9215) (-14.3029, -7.9215) (-14.7105, -7.3751) (-14.7105, -6.8255) knots 0 0 0 1 2 2 2
  line L178 (-17.2176, -5.9116) -> (-17.1929, -5.9116)
  spline S213 degree 2 poles (-17.1929, -5.9116) (-17.1373, -5.8961) (-17.0169, -5.89) (-16.9335, -5.89) knots 0 0 0 1 2 2 2
  spline S214 degree 2 poles (-16.9335, -5.89) (-16.739, -5.89) (-16.3561, -6.0598) (-16.1832, -6.2265) knots 0 0 0 1 2 2 2
  line L179 (-16.1832, -6.2265) -> (-16.1832, -8.255)
  line L180 (-16.1832, -8.255) -> (-15.7016, -8.255)
  line L181 (-15.7016, -8.255) -> (-15.7016, -5.396)
  line L182 (-15.7016, -5.396) -> (-16.1832, -5.396)
  line L183 (-16.1832, -5.396) -> (-16.1832, -5.822)
  spline S215 degree 2 poles (-16.1832, -5.822) (-16.4457, -5.5874) (-16.8378, -5.396) (-17.023, -5.396) knots 0 0 0 1 2 2 2
  spline S216 degree 2 poles (-17.023, -5.396) (-17.0971, -5.396) (-17.1712, -5.4021) (-17.2176, -5.4114) knots 0 0 0 1 2 2 2
  line L184 (-17.2176, -5.4114) -> (-17.2176, -5.9116)
  line L185 (-20.833, -8.255) -> (-20.833, -6.6001)
  spline S217 degree 2 poles (-20.833, -6.6001) (-20.833, -6.4025) (-20.8022, -6.0659) (-20.7528, -5.9733) knots 0 0 0 1 2 2 2
  spline S218 degree 2 poles (-20.7528, -5.9733) (-20.7034, -5.8714) (-20.515, -5.7726) (-20.3514, -5.7726) knots 0 0 0 1 2 2 2
  spline S219 degree 2 poles (-20.3514, -5.7726) (-20.2032, -5.7726) (-19.8636, -5.9548) (-19.6845, -6.1277) knots 0 0 0 1 2 2 2
  spline S220 degree 2 poles (-19.6845, -6.1277) (-19.6876, -6.1709) (-19.6937, -6.2913) (-19.6937, -6.3716) knots 0 0 0 1 2 2 2
  line L186 (-19.6937, -6.3716) -> (-19.6937, -8.255)
  line L187 (-19.6937, -8.255) -> (-19.2121, -8.255)
  line L188 (-19.2121, -8.255) -> (-19.2121, -6.6001)
  spline S221 degree 2 poles (-19.2121, -6.6001) (-19.2121, -6.4025) (-19.1812, -6.0659) (-19.1318, -5.9733) knots 0 0 0 1 2 2 2
  spline S222 degree 2 poles (-19.1318, -5.9733) (-19.0824, -5.8714) (-18.8941, -5.7726) (-18.7304, -5.7726) knots 0 0 0 1 2 2 2
  spline S223 degree 2 poles (-18.7304, -5.7726) (-18.5761, -5.7726) (-18.2333, -5.9671) (-18.0728, -6.1184) knots 0 0 0 1 2 2 2
  line L189 (-18.0728, -6.1184) -> (-18.0728, -8.255)
  line L190 (-18.0728, -8.255) -> (-17.5911, -8.255)
  line L191 (-17.5911, -8.255) -> (-17.5911, -5.396)
  line L192 (-17.5911, -5.396) -> (-18.0728, -5.396)
  line L193 (-18.0728, -5.396) -> (-18.0728, -5.7109)
  spline S224 degree 2 poles (-18.0728, -5.7109) (-18.2611, -5.5225) (-18.6316, -5.3157) (-18.8539, -5.3157) knots 0 0 0 1 2 2 2
  spline S225 degree 2 poles (-18.8539, -5.3157) (-19.1071, -5.3157) (-19.4992, -5.5472) (-19.6011, -5.8097) knots 0 0 0 1 2 2 2
  spline S226 degree 2 poles (-19.6011, -5.8097) (-19.8203, -5.5658) (-20.2341, -5.3157) (-20.4749, -5.3157) knots 0 0 0 1 2 2 2
  spline S227 degree 2 poles (-20.4749, -5.3157) (-20.6601, -5.3157) (-20.9627, -5.4299) (-21.0739, -5.5596) knots 0 0 0 1 2 2 2
  spline S228 degree 2 poles (-21.0739, -5.5596) (-21.1881, -5.6893) (-21.3147, -6.0783) (-21.3147, -6.3716) knots 0 0 0 1 2 2 2
  line L194 (-21.3147, -6.3716) -> (-21.3147, -8.255)
  line L195 (-21.3147, -8.255) -> (-20.833, -8.255)
  spline S229 degree 2 poles (-23.6242, -8.3291) (-23.2197, -8.3291) (-22.5497, -8.0821) (-22.3089, -7.832) knots 0 0 0 1 2 2 2
  spline S230 degree 2 poles (-22.3089, -7.832) (-22.068, -7.5788) (-21.8118, -6.8317) (-21.8118, -6.3469) knots 0 0 0 1 2 2 2
  spline S231 degree 2 poles (-21.8118, -6.3469) (-21.8118, -5.8869) (-22.0711, -5.1582) (-22.312, -4.8989) knots 0 0 0 1 2 2 2
  spline S232 degree 2 poles (-22.312, -4.8989) (-22.5435, -4.6488) (-23.2228, -4.3771) (-23.6272, -4.3771) knots 0 0 0 1 2 2 2
  spline S233 degree 2 poles (-23.6272, -4.3771) (-23.8218, -4.3771) (-24.1737, -4.4326) (-24.3343, -4.4821) knots 0 0 0 1 2 2 2
  spline S234 degree 2 poles (-24.3343, -4.4821) (-24.464, -4.5191) (-24.7789, -4.655) (-24.8746, -4.7044) knots 0 0 0 1 2 2 2
  line L196 (-24.8746, -4.7044) -> (-24.8746, -5.3157)
  line L197 (-24.8746, -5.3157) -> (-24.8314, -5.3157)
  spline S235 degree 2 poles (-24.8314, -5.3157) (-24.7357, -5.2323) (-24.535, -5.081) (-24.3497, -4.9946) knots 0 0 0 1 2 2 2
  spline S236 degree 2 poles (-24.3497, -4.9946) (-24.1954, -4.9174) (-23.7971, -4.8155) (-23.5686, -4.8155) knots 0 0 0 1 2 2 2
  spline S237 degree 2 poles (-23.5686, -4.8155) (-23.019, -4.8155) (-22.3398, -5.643) (-22.3398, -6.3315) knots 0 0 0 1 2 2 2
  spline S238 degree 2 poles (-22.3398, -6.3315) (-22.3398, -6.7143) (-22.5188, -7.2886) (-22.6886, -7.4862) knots 0 0 0 1 2 2 2
  spline S239 degree 2 poles (-22.6886, -7.4862) (-22.8523, -7.6838) (-23.3154, -7.8907) (-23.6056, -7.8907) knots 0 0 0 1 2 2 2
  spline S240 degree 2 poles (-23.6056, -7.8907) (-23.8187, -7.8907) (-24.2448, -7.8289) (-24.3899, -7.7672) knots 0 0 0 1 2 2 2
  line L198 (-24.3899, -7.7672) -> (-24.3899, -6.7823)
  line L199 (-24.3899, -6.7823) -> (-23.5068, -6.7823)
  line L200 (-23.5068, -6.7823) -> (-23.5068, -6.3376)
  line L201 (-23.5068, -6.3376) -> (-24.89, -6.3376)
  line L202 (-24.89, -6.3376) -> (-24.89, -8.0018)
  spline S241 degree 2 poles (-24.89, -8.0018) (-24.7943, -8.045) (-24.4671, -8.1778) (-24.3281, -8.2179) knots 0 0 0 1 2 2 2
  spline S242 degree 2 poles (-24.3281, -8.2179) (-24.1398, -8.2735) (-23.8372, -8.3291) (-23.6242, -8.3291) knots 0 0 0 1 2 2 2
  spline S243 degree 2 poles (-26.7302, -8.3198) (-26.0448, -8.3198) (-25.2914, -7.551) (-25.2914, -6.8409) knots 0 0 0 1 2 2 2
  spline S244 degree 2 poles (-25.2914, -6.8409) (-25.2914, -6.1431) (-26.0232, -5.3157) (-26.6129, -5.3157) knots 0 0 0 1 2 2 2
  spline S245 degree 2 poles (-26.6129, -5.3157) (-26.8784, -5.3157) (-27.289, -5.4701) (-27.4403, -5.6337) knots 0 0 0 1 2 2 2
  spline S246 degree 2 poles (-27.4403, -5.6337) (-27.5947, -5.7973) (-27.7583, -6.2697) (-27.7583, -6.6124) knots 0 0 0 1 2 2 2
  line L203 (-27.7583, -6.6124) -> (-27.7583, -6.8749)
  line L204 (-27.7583, -6.8749) -> (-25.7792, -6.8749)
  spline S247 degree 2 poles (-25.7792, -6.8749) (-25.7792, -7.372) (-26.2794, -7.8999) (-26.724, -7.8999) knots 0 0 0 1 2 2 2
  spline S248 degree 2 poles (-26.724, -7.8999) (-26.8815, -7.8999) (-27.1872, -7.8289) (-27.3107, -7.7733) knots 0 0 0 1 2 2 2
  spline S249 degree 2 poles (-27.3107, -7.7733) (-27.4403, -7.7116) (-27.6194, -7.6035) (-27.6781, -7.5541) knots 0 0 0 1 2 2 2
  line L205 (-27.6781, -7.5541) -> (-27.7059, -7.5541)
  line L206 (-27.7059, -7.5541) -> (-27.7059, -8.079)
  spline S250 degree 2 poles (-27.7059, -8.079) (-27.6225, -8.113) (-27.3693, -8.2118) (-27.2705, -8.2396) knots 0 0 0 1 2 2 2
  spline S251 degree 2 poles (-27.2705, -8.2396) (-27.1316, -8.2797) (-26.9031, -8.3198) (-26.7302, -8.3198) knots 0 0 0 1 2 2 2
  spline S252 degree 2 poles (-27.289, -6.5075) (-27.2829, -6.3129) (-27.2026, -6.0289) (-27.1254, -5.9332) knots 0 0 0 1 2 2 2
  spline S253 degree 2 poles (-27.1254, -5.9332) (-27.042, -5.8251) (-26.7796, -5.7109) (-26.5851, -5.7109) knots 0 0 0 1 2 2 2
  spline S254 degree 2 poles (-26.5851, -5.7109) (-26.3937, -5.7109) (-26.1251, -5.8251) (-26.0139, -5.9363) knots 0 0 0 1 2 2 2
  spline S255 degree 2 poles (-26.0139, -5.9363) (-25.9058, -6.0505) (-25.7947, -6.3253) (-25.7792, -6.5075) knots 0 0 0 1 2 2 2
  line L207 (-25.7792, -6.5075) -> (-27.289, -6.5075)
  spline S256 degree 2 poles (-29.8393, -7.9524) (-29.7807, -7.9956) (-29.5831, -8.15) (-29.4904, -8.1963) knots 0 0 0 1 2 2 2
  spline S257 degree 2 poles (-29.4904, -8.1963) (-29.3639, -8.2643) (-29.1261, -8.3353) (-28.91, -8.3353) knots 0 0 0 1 2 2 2
  spline S258 degree 2 poles (-28.91, -8.3353) (-28.734, -8.3353) (-28.416, -8.2025) (-28.2956, -8.0821) knots 0 0 0 1 2 2 2
  spline S259 degree 2 poles (-28.2956, -8.0821) (-28.1813, -7.9648) (-28.0424, -7.619) (-28.0424, -7.4275) knots 0 0 0 1 2 2 2
  spline S260 degree 2 poles (-28.0424, -7.4275) (-28.0424, -7.1311) (-28.2925, -6.7112) (-28.5642, -6.5908) knots 0 0 0 1 2 2 2
  spline S261 degree 2 poles (-28.5642, -6.5908) (-28.805, -6.4797) (-29.4596, -6.3963) (-29.8393, -6.3747) knots 0 0 0 1 2 2 2
  line L208 (-29.8393, -6.3747) -> (-29.8393, -6.2821)
  spline S262 degree 2 poles (-29.8393, -6.2821) (-29.8393, -6.1153) (-29.7375, -5.9085) (-29.6448, -5.8498) knots 0 0 0 1 2 2 2
  spline S263 degree 2 poles (-29.6448, -5.8498) (-29.5522, -5.7912) (-29.2867, -5.7541) (-29.1446, -5.7541) knots 0 0 0 1 2 2 2
  spline S264 degree 2 poles (-29.1446, -5.7541) (-28.9779, -5.7541) (-28.5271, -5.8529) (-28.3018, -5.9486) knots 0 0 0 1 2 2 2
  line L209 (-28.3018, -5.9486) -> (-28.274, -5.9486)
  line L210 (-28.274, -5.9486) -> (-28.274, -5.4577)
  spline S265 degree 2 poles (-28.274, -5.4577) (-28.4067, -5.4207) (-28.9038, -5.328) (-29.1477, -5.328) knots 0 0 0 1 2 2 2
  spline S266 degree 2 poles (-29.1477, -5.328) (-29.4441, -5.328) (-29.8486, -5.4207) (-30.0092, -5.5411) knots 0 0 0 1 2 2 2
  spline S267 degree 2 poles (-30.0092, -5.5411) (-30.1666, -5.6584) (-30.321, -6.032) (-30.321, -6.3006) knots 0 0 0 1 2 2 2
  line L211 (-30.321, -6.3006) -> (-30.321, -8.255)
  line L212 (-30.321, -8.255) -> (-29.8393, -8.255)
  line L213 (-29.8393, -8.255) -> (-29.8393, -7.9524)
  line L214 (-29.8393, -7.551) -> (-29.8393, -6.7576)
  spline S268 degree 2 poles (-29.8393, -6.7576) (-29.6664, -6.773) (-29.1446, -6.8255) (-28.981, -6.8749) knots 0 0 0 1 2 2 2
  spline S269 degree 2 poles (-28.981, -6.8749) (-28.7896, -6.9335) (-28.5395, -7.1775) (-28.5395, -7.3936) knots 0 0 0 1 2 2 2
  spline S270 degree 2 poles (-28.5395, -7.3936) (-28.5395, -7.6406) (-28.8174, -7.8907) (-29.0829, -7.8907) knots 0 0 0 1 2 2 2
  spline S271 degree 2 poles (-29.0829, -7.8907) (-29.3083, -7.8907) (-29.6788, -7.6962) (-29.8393, -7.551) knots 0 0 0 1 2 2 2
  line L215 (-32.5131, -5.9116) -> (-32.4884, -5.9116)
  spline S272 degree 2 poles (-32.4884, -5.9116) (-32.4329, -5.8961) (-32.3124, -5.89) (-32.2291, -5.89) knots 0 0 0 1 2 2 2
  spline S273 degree 2 poles (-32.2291, -5.89) (-32.0346, -5.89) (-31.6517, -6.0598) (-31.4788, -6.2265) knots 0 0 0 1 2 2 2
  line L216 (-31.4788, -6.2265) -> (-31.4788, -8.255)
  line L217 (-31.4788, -8.255) -> (-30.9972, -8.255)
  line L218 (-30.9972, -8.255) -> (-30.9972, -5.396)
  line L219 (-30.9972, -5.396) -> (-31.4788, -5.396)
  line L220 (-31.4788, -5.396) -> (-31.4788, -5.822)
  spline S274 degree 2 poles (-31.4788, -5.822) (-31.7413, -5.5874) (-32.1334, -5.396) (-32.3186, -5.396) knots 0 0 0 1 2 2 2
  spline S275 degree 2 poles (-32.3186, -5.396) (-32.3927, -5.396) (-32.4668, -5.4021) (-32.5131, -5.4114) knots 0 0 0 1 2 2 2
  line L221 (-32.5131, -5.4114) -> (-32.5131, -5.9116)
  line L222 (-37.3235, -4.445) -> (-36.0113, -8.255)
  line L223 (-36.0113, -8.255) -> (-35.4648, -8.255)
  line L224 (-35.4648, -8.255) -> (-34.1526, -4.445)
  line L225 (-34.1526, -4.445) -> (-34.696, -4.445)
  line L226 (-34.696, -4.445) -> (-35.7519, -7.6097)
  line L227 (-35.7519, -7.6097) -> (-36.8079, -4.445)
  line L228 (-36.8079, -4.445) -> (-37.3235, -4.445)
  spline S276 degree 2 poles (-39.9942, -6.35) (-39.9942, -7.3751) (-39.3983, -8.3353) (-38.7777, -8.3353) knots 0 0 0 1 2 2 2
  spline S277 degree 2 poles (-38.7777, -8.3353) (-38.1479, -8.3353) (-37.5581, -7.3565) (-37.5581, -6.3531) knots 0 0 0 1 2 2 2
  spline S278 degree 2 poles (-37.5581, -6.3531) (-37.5581, -5.3219) (-38.154, -4.3678) (-38.7777, -4.3678) knots 0 0 0 1 2 2 2
  spline S279 degree 2 poles (-38.7777, -4.3678) (-39.4045, -4.3678) (-39.9942, -5.3558) (-39.9942, -6.35) knots 0 0 0 1 2 2 2
  spline S280 degree 2 poles (-39.3396, -7.5109) (-39.4137, -7.3226) (-39.4755, -6.7421) (-39.4755, -6.35) knots 0 0 0 1 2 2 2
  spline S281 degree 2 poles (-39.4755, -6.35) (-39.4755, -5.9579) (-39.4137, -5.3805) (-39.3366, -5.186) knots 0 0 0 1 2 2 2
  spline S282 degree 2 poles (-39.3366, -5.186) (-39.2594, -4.9915) (-38.9907, -4.7908) (-38.7777, -4.7908) knots 0 0 0 1 2 2 2
  spline S283 degree 2 poles (-38.7777, -4.7908) (-38.5647, -4.7908) (-38.2899, -4.9915) (-38.2096, -5.1922) knots 0 0 0 1 2 2 2
  spline S284 degree 2 poles (-38.2096, -5.1922) (-38.1324, -5.3867) (-38.0768, -5.9795) (-38.0768, -6.3531) knots 0 0 0 1 2 2 2